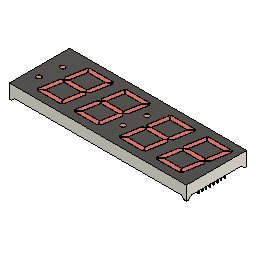
1.2in 7 Segment Display (Autodesk Fusion 360 design; units mm, degrees)
Autodesk Fusion 360 part; units mm, degrees
note: some values were not read from the file. Chosen so that the rebuilt part matches the saved one: which bodies a step acts on.
sketch "base" plane through (0, 0, 0) normal (0, 0, 1) x (1, 0, 0)
  line L0 (-60, 20.4) -> (60, 20.4)
  line L1 (60, 20.4) -> (60, -20.4)
  line L2 (60, -20.4) -> (-60, -20.4)
  line L3 (-60, -20.4) -> (-60, 20.4)
  line L4 (0, 20.4) -> (0, 0) construction
  line L5 (0, 0) -> (-60, 0) construction
  dimension "d1" = 120
  dimension "d2" = 40.8
  constraint horizontal L0
  constraint vertical L1
  constraint horizontal L2
  constraint vertical L3
  constraint midpoint L0 L4.start
  constraint perpendicular L0 L4
  constraint perpendicular L4 L5
  constraint midpoint L3 L5.end
  constraint coincident L4.end L5.start
  measures "d1" distance of L0.start L0.end
  measures "d2" distance of L0.end L1.end
extrude "Extrude1" add sketch "base" along normal blind 9.5 makes body 1
sketch "y cuts" plane through (0, 0, 0) normal (1, 0, 0) x (0, 1, 0)
  line L0 (-19, 0) -> (19, 0)
  line L1 (19, 0) -> (17, 2)
  line L2 (17, 2) -> (-17, 2)
  line L3 (-17, 2) -> (-19, 0)
  dimension "d5" = 38
  dimension "d6" = 45
  dimension "d7" = 2
  constraint horizontal L0
  constraint parallel L0 L2
  constraint coincident L0.start L3.end
  constraint equal L1 L3
  constraint midpoint origin L0
  measures "d5" distance of L0.start L0.end
  measures "d6" angle of L0 L1
  measures "d7" distance of L0 L2
extrude "Extrude2" cut sketch "y cuts" along normal through all and the other way through all bodies 1
sketch "x cuts" plane through (0, 0, 0) normal (0, 1, 0) x (1, 0, 0)
  line L0 (-58.5, 0) -> (58.5, 0)
  line L1 (58.5, 0) -> (56.5, -2)
  line L2 (56.5, -2) -> (-56.5, -2)
  line L3 (-56.5, -2) -> (-58.5, 0)
  dimension "d9" = 45
  dimension "d10" = 2
  dimension "d11" = 117
  constraint horizontal L0
  constraint parallel L0 L2
  constraint equal L1 L3
  constraint midpoint origin L0
  measures "d9" angle of L0 L3
  measures "d10" distance of L0 L2
  measures "d11" distance of L0.start L0.end
extrude "Extrude3" cut sketch "x cuts" along normal through all and the other way through all bodies 1
sketch "pins" plane through (0, 0, 0) normal (0, 0, 1) x (1, 0, 0)
  line L0 (55.2, 10.46) -> (55.8, 10.46)
  line L1 (55.8, 10.46) -> (55.8, 9.86)
  line L2 (55.8, 9.86) -> (55.2, 9.86)
  line L3 (55.2, 9.86) -> (55.2, 10.46)
  line L4 (55.5, 10.46) -> (55.5, 10.16) construction
  line L5 (55.5, 10.16) -> (55.2, 10.16) construction
  line L6 (55.2, 7.92) -> (55.8, 7.92)
  line L7 (55.8, 7.92) -> (55.8, 7.32)
  line L8 (55.8, 7.32) -> (55.2, 7.32)
  line L9 (55.2, 7.32) -> (55.2, 7.92)
  line L10 (55.2, 5.38) -> (55.8, 5.38)
  line L11 (55.8, 5.38) -> (55.8, 4.78)
  line L12 (55.8, 4.78) -> (55.2, 4.78)
  line L13 (55.2, 4.78) -> (55.2, 5.38)
  line L14 (55.2, 2.84) -> (55.8, 2.84)
  line L15 (55.8, 2.84) -> (55.8, 2.24)
  line L16 (55.8, 2.24) -> (55.2, 2.24)
  line L17 (55.2, 2.24) -> (55.2, 2.84)
  line L18 (55.2, 0.3) -> (55.8, 0.3)
  line L19 (55.8, 0.3) -> (55.8, -0.3)
  line L20 (55.8, -0.3) -> (55.2, -0.3)
  line L21 (55.2, -0.3) -> (55.2, 0.3)
  line L22 (55.2, -2.24) -> (55.8, -2.24)
  line L23 (55.8, -2.24) -> (55.8, -2.84)
  line L24 (55.8, -2.84) -> (55.2, -2.84)
  line L25 (55.2, -2.84) -> (55.2, -2.24)
  line L26 (55.2, -4.78) -> (55.8, -4.78)
  line L27 (55.8, -4.78) -> (55.8, -5.38)
  line L28 (55.8, -5.38) -> (55.2, -5.38)
  line L29 (55.2, -5.38) -> (55.2, -4.78)
  line L30 (55.2, -7.32) -> (55.8, -7.32)
  line L31 (55.8, -7.32) -> (55.8, -7.92)
  line L32 (55.8, -7.92) -> (55.2, -7.92)
  line L33 (55.2, -7.92) -> (55.2, -7.32)
  dimension "d13" = 0.6
  dimension "d14" = 0.6
  dimension "d15" = 55.5
  dimension "d16" = 10.16
  dimension "d19" = 0
  dimension "d20" = -2.54
  constraint horizontal L0
  constraint vertical L1
  constraint horizontal L2
  constraint vertical L3
  constraint midpoint L0 L4.start
  constraint perpendicular L0 L4
  constraint midpoint L3 L5.end
  constraint perpendicular L3 L5
  measures "d13" distance of L0.start L0.end
  measures "d14" distance of L0.start L2.end
  measures "d15" distance of origin L4
  measures "d16" distance of origin L5
extrude "Extrude4" add sketch "pins" along normal blind -4 and the other way up to surface (-2 mm away) separate body makes body 2 at (55.2, 4.98, 0) makes body 3 at (55.2, -5.18, 0) makes body 4 at (55.2, -2.64, 0) makes body 5 at (55.2, 7.52, 0) makes body 6 at (55.2, 2.44, 0) makes body 7 at (55.2, -7.72, 0) makes body 8 at (55.2, -0.1, 0) makes body 9 at (55.2, 10.06, 0)
mirror "Mirror1" about plane through (0, 0, 0) normal (1, 0, 0) of bodies 9 8 7 6 5 4 3 2 makes body 10 at (-55.2, 4.98, 0) makes body 11 at (-55.2, -5.18, 0) makes body 12 at (-55.2, -2.64, 0) makes body 13 at (-55.2, 7.52, 0) makes body 14 at (-55.2, 2.44, 0) makes body 15 at (-55.2, -7.72, 0) makes body 16 at (-55.2, -0.1, 0) makes body 17 at (-55.2, 10.06, 0)
ref_plane "WorkPlane1" through (0, 0, 9.5) normal (0, 0, 1) x (1, 0, 0)
sketch "digits" plane through (0, 0, 9.5) normal (0, 0, 1) x (1, 0, 0)
  line L0 (-41.9358, 15.3) -> (-24.0642, 15.3)
  line L1 (-24.0642, 15.3) -> (-29.4599, -15.3)
  line L2 (-29.4599, -15.3) -> (-47.3314, -15.3)
  line L3 (-47.3314, -15.3) -> (-41.9358, 15.3)
  line L4 (-33, 15.3) -> (-33, 0) construction
  line L5 (-33, 0) -> (-44.6336, 0) construction
  circle A0 centre (-51.0337, 6.8937) radius 1.5
  line L6 (-51.0337, 6.8937) -> (-53.4648, -6.8937) construction
  circle A1 centre (-53.4648, -6.8937) radius 1.5
  line L7 (-52.2493, 0) -> (-44.6336, 0) construction
  line L8 (-47.0929, -13.9475) -> (-45.7404, -15.3)
  line L9 (-30.7815, -15.3) -> (-29.2304, -13.9985)
  line L10 (-25.2024, 15.3) -> (-24.2932, 14.0015)
  line L11 (-41.0913, 15.3) -> (-42.0824, 14.4683)
  dimension "d28" = 30.6
  dimension "d29" = 17.6
  dimension "d34" = 33
  dimension "d35" = 10
  dimension "d36" = 3
  dimension "d37" = 7.5
  dimension "d38" = 14
  dimension "d67" = 45
  dimension "d69" = 40
  dimension "d70" = 45
  dimension "d71" = 40
  constraint horizontal L0
  constraint parallel L0 L2
  constraint parallel L1 L3
  constraint midpoint L0 L4.start
  constraint perpendicular L0 L4
  constraint perpendicular L4 L5
  constraint midpoint L3 L5.end
  constraint coincident origin L5
  constraint coincident A0.centre L6.start
  constraint parallel L3 L6
  constraint coincident L6.end A1.centre
  constraint equal A0 A1
  constraint midpoint L6 L7.start
  constraint horizontal L7
  constraint coincident L3 L8.start
  constraint coincident L2 L8.end
  constraint coincident L2 L9.start
  constraint coincident L1 L9.end
  constraint coincident L0 L10.start
  constraint coincident L1 L10.end
  constraint coincident L0 L11.start
  constraint coincident L3 L11.end
  measures "d28" distance of L0 L2
  measures "d29" distance of L1 L3
  measures "d34" distance of origin L4
  measures "d35" angle of L1 L4
  measures "d36" diameter of A0
  measures "d37" distance of L3 L6
  measures "d38" distance of A0.centre L6.end
  measures "d67" angle of L2 L8
  measures "d69" angle of L1 L9
  measures "d70" angle of L1 L10
  measures "d71" angle of L3 L11
extrude "Extrude5" add sketch "digits" along normal blind 0.2 separate body contours A0 | A1 makes body 18 at (-51.4058, 7.1592, 9.5) makes body 19 at (-53.8369, -6.6281, 9.5)
extrude "Extrude6" add sketch "digits" along normal blind 0.2 separate body contours L0 L3 L11 | L0 L1 L2 L3 L8 L9 L10 L11 | L0 L1 L10 | L2 L3 L8 | L1 L2 L9 makes body 20
shell "Shell1" thickness 3 removed faces 2 at (-39.5757, -5.1, 9.7) at (-39.5757, -5.1, 9.5) on bodies 20
sketch "digit cuts" plane through (0, 0, 9.7) normal (0, 0, 1) x (-1, 0, 0)
  line L0 (43.7561, 12.3) -> (39.4185, -12.3)
  line L1 (39.4185, -12.3) -> (27.6395, -12.3)
  line L2 (27.6395, -12.3) -> (31.9772, 12.3)
  line L3 (31.9772, 12.3) -> (43.7561, 12.3)
  line L4 (47.3314, 15.3) -> (29.4599, 15.3)
  line L5 (29.4599, 15.3) -> (24.0642, -15.3)
  line L6 (24.0642, -15.3) -> (41.9358, -15.3)
  line L7 (41.9358, -15.3) -> (47.3314, 15.3)
  line L8 (44.6336, 0) -> (26.762, 0)
  line L9 (42.1709, -15.5802) -> (37.0392, -9.4645)
  line L10 (28.474, -11.5998) -> (22.3583, -16.7314)
  line L11 (32.2223, 12.0078) -> (27.0522, 18.1693)
  line L12 (48.5821, 16.3495) -> (42.1006, 10.9109)
  line L13 (41.6225, 0.2) -> (44.6688, 0.2) construction
  line L14 (44.5983, -0.2) -> (41.552, -0.2) construction
  line L15 (43.0752, -0.2) -> (44.3338, -1.7)
  line L16 (43.0752, -0.2) -> (41.2875, -1.7)
  line L17 (44.3338, -1.7) -> (41.2875, -1.7) construction
  line L18 (44.9333, 1.7) -> (43.1457, 0.2)
  line L19 (43.1457, 0.2) -> (41.887, 1.7)
  line L20 (41.887, 1.7) -> (44.9333, 1.7) construction
  line L21 (29.7731, -0.2) -> (26.7268, -0.2) construction
  line L22 (29.8436, 0.2) -> (26.7973, 0.2) construction
  line L23 (30.1081, 1.7) -> (28.3205, 0.2)
  line L24 (28.3205, 0.2) -> (27.0618, 1.7)
  line L25 (30.1081, 1.7) -> (27.0618, 1.7) construction
  line L26 (29.5086, -1.7) -> (26.4623, -1.7) construction
  line L27 (26.4623, -1.7) -> (28.2499, -0.2)
  line L28 (28.2499, -0.2) -> (29.5086, -1.7)
  dimension "d52" = 0.2
  dimension "d53" = 0.2
  dimension "d56" = 0.2
  dimension "d57" = 0.2
  constraint midpoint L7 L8.start
  constraint midpoint L5 L8.end
  constraint coincident L0.end L9
  constraint coincident L6.end L9
  constraint coincident L5.end L10
  constraint coincident L1.end L10
  constraint equal L9 L10
  constraint coincident L4.end L11
  constraint coincident L2.end L11
  constraint coincident L0.start L12
  constraint coincident L4.start L12
  constraint coincident L7 L13.end
  constraint coincident L0 L13.start
  constraint horizontal L13
  constraint coincident L0 L14.end
  constraint coincident L7 L14.start
  constraint horizontal L14
  constraint midpoint L14 L15.start
  constraint coincident L7 L15.end
  constraint coincident L0 L16.end
  constraint horizontal L17
  constraint coincident L7 L18.start
  constraint coincident L13 L18.end
  constraint perpendicular L18 L19
  constraint coincident L0 L19.end
  constraint horizontal L20
  constraint coincident L2 L21.start
  constraint coincident L5 L21.end
  constraint parallel L8 L21
  constraint coincident L2 L22.start
  constraint coincident L5 L22.end
  constraint horizontal L22
  constraint perpendicular L23 L24
  constraint horizontal L25
  constraint midpoint L22 L23.end
  constraint coincident L5 L24.end
  constraint coincident L2 L23.start
  constraint midpoint L13 L18.end
  constraint perpendicular L15 L16
  constraint horizontal L26
  constraint perpendicular L27 L28
  constraint coincident L26.start L28.end
  constraint midpoint L21 L27.end
  constraint coincident L5 L26.end
  constraint coincident L2 L26.start
  measures "d52" distance of L8 L13
  measures "d53" distance of L8 L14
  measures "d56" distance of L8 L21
  measures "d57" distance of L8 L22
extrude "Extrude8" cut sketch "digit cuts" against normal blind 2 thin wall 0.4 centred open curves L10 L9 L12 L11 bodies 20 makes body 21 at (-31.3336, 14.3, 9.5) makes body 22 at (-27.0754, 3.9814, 9.5) makes body 23 at (-40.062, -14.3, 9.5)
extrude "Extrude13" cut sketch "digits" along normal blind 2 contours L0 L3 L11 | L0 L1 L10 | L2 L3 L8 | L1 L2 L9 bodies 20 21 22 23
extrude "Extrude10" cut sketch "digit cuts" against normal blind 2 contours L0 L7 L8 L18 L19 | L0 L7 L8 L15 L16 | L2 L5 L8 L23 L24 | L2 L5 L8 L27 L28 bodies 20 makes body 24 at (-41.96, 9.4037, 9.5)
extrude "Extrude11" cut sketch "digit cuts" against normal blind 2 contours L2 L5 L8 L23 L24 | L2 L5 L8 L27 L28 bodies 22 makes body 25 at (-29.408, -9.2471, 9.7)
sketch "digit middle" plane through (0, 0, 9.5) normal (0, 0, 1) x (1, 0, 0)
  line L0 (-42.6912, 0) -> (-28.6043, 0) construction
  line L1 (-42.6912, 0) -> (-40.9036, 1.5)
  line L2 (-40.9036, 1.5) -> (-29.8629, 1.5)
  line L3 (-42.6912, 0) -> (-41.4326, -1.5)
  line L4 (-41.4326, -1.5) -> (-30.3919, -1.5)
  line L5 (-43.0752, 0.2) -> (-41.2875, 1.7)
  line L6 (-41.887, -1.7) -> (-43.1457, -0.2)
  line L7 (-29.8629, 1.5) -> (-28.6043, 0)
  line L8 (-30.3919, -1.5) -> (-28.6043, 0)
  line L9 (-29.5086, 1.7) -> (-28.2499, 0.2)
  line L10 (-28.3205, -0.2) -> (-30.1081, -1.7)
  dimension "d60" = 1.5
  dimension "d61" = 1.5
  dimension "d62" = 0.4
  dimension "d63" = 0.4
  constraint horizontal L0
  constraint parallel L0 L2
  constraint horizontal L4
  constraint coincident origin L0
  constraint parallel L1 L5
  constraint parallel L3 L6
  constraint parallel L8 L10
  constraint parallel L7 L9
  measures "d60" distance of L0 L4
  measures "d61" distance of L0 L2
  measures "d62" distance of L1 L5
  measures "d63" distance of L7 L9
extrude "Extrude12" add sketch "digit middle" along normal blind 0.2 separate body makes body 26
copy_body "CopyPasteBodies2" bodies 26 25 24 23 22 21 20 makes body 27 makes body 28 makes body 29 makes body 30 makes body 31 makes body 32 makes body 33
move_body "Move2" bodies 27 28 29 30 31 32 33 to x (1, 0, 0) y (0, 1, 0) z (0, 0, 1) at (25, 0, 0)
copy_body "CopyPasteBodies3" bodies 27 33 31 32 29 30 28 makes body 34 makes body 35 makes body 36 makes body 37 makes body 38 makes body 39 makes body 40
move_body "Move3" bodies 34 35 36 37 38 39 40 to x (1, 0, 0) y (0, 1, 0) z (0, 0, 1) at (30.6, 0, 0)
copy_body "CopyPasteBodies4" bodies 40 34 37 35 39 36 38 makes body 41 makes body 42 makes body 43 makes body 44 makes body 45 makes body 46 makes body 47
move_body "Move4" bodies 41 42 43 44 45 46 47 to x (1, 0, 0) y (0, 1, 0) z (0, 0, 1) at (25, 0, 0)
copy_body "CopyPasteBodies5" bodies 19 18 makes body 48 makes body 49
move_body "Move5" bodies 48 49 to x (1, 0, 0) y (0, 1, 0) z (0, 0, 1) at (57, 0, 0)
equation "d15 = ( 111 / 2 ) * 1 mm"
equation "d16 = 20.32 mm / 2"
named bodies: "dot 1", "dot 2", "digit 1", "digit 2", "digit 3", "digit 4", "digit 5", "digit 6", "digit 7", "digit 7 (1)", "digit 6 (1)", "digit 5 (1)", "digit 4 (1)", "digit 3 (1)", "digit 2 (1)", "digit 1 (1)", "digit 7 (1) (1)", "digit 1 (1) (1)", "digit 3 (1) (1)", "digit 2 (1) (1)", "digit 5 (1) (1)", "digit 4 (1) (1)", "digit 6 (1) (1)", "digit 6 (1) (1) (1)", "digit 7 (1) (1) (1)", "digit 2 (1) (1) (1)", "digit 1 (1) (1) (1)", "digit 4 (1) (1) (1)", "digit 3 (1) (1) (1)", "digit 5 (1) (1) (1)", "dot 2 (1)", "dot 1 (1)"
